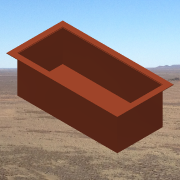
# Autodesk Inventor part: dcps_mcpc
Saved by Autodesk Inventor 2014 SP1 (Build 180222100, 222)
## iProperties
Created: 2014-03-12
Part Number: dcps_mcpc
Material: Copper, Alloy
Document SubType Name: Modeling
Designer: Dave
Density: 7.58 g/cm^3
Appearance: Copper - Satin
Mass: 372642 g
Surface Area: 8387.08 cm^2
Volume: 49161.2 cm^3
Author: Dave
Autodesk Inventor part; units mm, degrees
ref_plane "YZ Plane" through (0, 0, 0) normal (1, 0, 0) x (0, 1, 0)
ref_plane "XZ Plane" through (0, 0, 0) normal (0, 1, 0) x (-1, 0, 0)
ref_plane "XY Plane" through (0, 0, 0) normal (0, 0, 1) x (1, 0, 0)
sketch "Sketch1" plane through (0, 0, 0) normal (0, 1, 0) x (-1, 0, 0)
  line L0 (-279.4, -127) -> (279.4, -127)
  line L1 (279.4, -127) -> (279.4, 127)
  line L2 (279.4, 127) -> (-279.4, 127)
  line L3 (-279.4, 127) -> (-279.4, -127)
  line L4 (-279.4, -127) -> (279.4, 127) construction
  line L5 (279.4, -127) -> (-279.4, 127) construction
  point P0 (0, 0)
  dimension "d0" = 558.8
  dimension "d1" = 254
  constraints: 12 end point, 2 midpoint, 2 parallel, 1 horizontal, 1 perpendicular
  measures "d0" distance of L2.end L1.end
  measures "d1" distance of L1.end L0.end
extrude "Extrusion1" add sketch "Sketch1" along normal blind 203.2
sketch "Sketch2" plane through (0, 203.2, 0) normal (0, 1, 0) x (1, 0, 0)
  line L0 (279.4, 127) -> (-279.4, 127) projected
  line L1 (-279.4, 127) -> (-279.4, -127) projected
  line L2 (-279.4, -127) -> (279.4, -127) projected
  line L3 (279.4, -127) -> (279.4, 127) projected
  line L4 (-309.4, 157) -> (309.4, 157)
  line L5 (309.4, 157) -> (309.4, -157)
  line L6 (309.4, -157) -> (-309.4, -157)
  line L7 (-309.4, -157) -> (-309.4, 157)
  point P0 (0, 0)
  dimension "d4" = 30
  constraints: 8 end point, 3 other
  measures "d4" distance between parallel lines of L0 L4
extrude "Extrusion2" add sketch "Sketch2" along normal blind 2.54
sketch "Sketch4" plane through (0, 203.2, 0) normal (0, 1, 0) x (1, 0, 0)
  line L0 (279.4, 127) -> (-279.4, 127) projected
  line L1 (-279.4, 127) -> (-279.4, -127) projected
  line L2 (-279.4, -127) -> (279.4, -127) projected
  line L3 (279.4, -127) -> (279.4, 127) projected
  line L4 (-276.86, 124.46) -> (276.86, 124.46)
  line L5 (276.86, 124.46) -> (276.86, -124.46)
  line L6 (276.86, -124.46) -> (-276.86, -124.46)
  line L7 (-276.86, -124.46) -> (-276.86, 124.46)
  point P0 (0, 0)
  dimension "d9" = 2.54
  constraints: 8 end point, 3 other
  measures "d9" distance between parallel lines of L4 L0
extrude "Extrusion4" cut sketch "Sketch4" against normal blind 175.26 contours L4 L5 L6 L7
body "Solid1"
